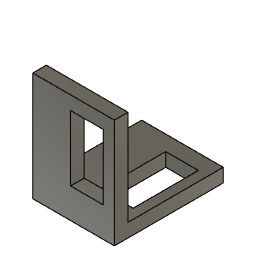
setSquare (Autodesk Fusion 360 design; units mm, degrees)
Autodesk Fusion 360 part; units mm, degrees
sketch "Esquisse1" plane through (0, 0, 0) normal (1, 0, 0) x (0, 1, 0)
  line L0 (0, 0) -> (40, 0)
  line L1 (0, 0) -> (0, 40)
  line L2 (0, 40) -> (5, 40)
  line L3 (5, 40) -> (5, 5)
  line L4 (5, 5) -> (40, 5)
  line L5 (40, 5) -> (40, 0)
  dimension "d2" = 40
  constraint coincident L0.start L1.start
  constraint horizontal L0
  constraint perpendicular L0 L1
  constraint perpendicular L1 L2
  constraint perpendicular L2 L3
  constraint perpendicular L3 L4
  constraint perpendicular L0 L5
  measures "d2" distance of L0.start L0.end
extrude "Extrusion1" add sketch "Esquisse1" along normal blind 30
sketch "Esquisse2" plane through (0, 0, 0) normal (0, 0, 1) x (1, 0, 0)
  line L0 (9.4451, 34.4261) -> (21.4451, 34.4261)
  line L1 (21.4451, 34.4261) -> (21.4451, 10.4261)
  line L2 (21.4451, 10.4261) -> (9.4451, 10.4261)
  line L3 (9.4451, 10.4261) -> (9.4451, 34.4261)
  dimension "d5" = 12
  dimension "d6" = 24
  constraint horizontal L0
  constraint vertical L1
  constraint horizontal L2
  constraint vertical L3
  measures "d5" distance of L0.start L0.end
  measures "d6" distance of L0.end L1.end
extrude "Extrusion2" cut sketch "Esquisse2" along normal blind 6
sketch "Esquisse4" plane through (0, 5, 0) normal (0, 1, 0) x (-1, 0, 0)
  line L0 (0, 5) -> (0, 40)
  line L1 (0, 40) -> (-30, 40)
  line L2 (-30, 40) -> (-30, 5)
  line L3 (-30, 5) -> (0, 5)
  line L4 (-8.8938, 10.999) -> (-20.8938, 10.999)
  line L5 (-20.8938, 10.999) -> (-20.8938, 34.999)
  line L6 (-20.8938, 34.999) -> (-8.8938, 34.999)
  line L7 (-8.8938, 34.999) -> (-8.8938, 10.999)
  dimension "d15" = 12
  dimension "d16" = 24
  constraint horizontal L4
  constraint vertical L5
  constraint horizontal L6
  constraint vertical L7
  measures "d15" distance of L4.start L4.end
  measures "d16" distance of L4.start L6.end
extrude "Extrusion3" cut sketch "Esquisse4" against normal blind 34 contours L4 L5 L6 L7
extrude "Extrusion4" cut 1 faces at (20.8938, 3.3333, 18.999) along direction (1, 0, 0) blind 5
extrude "Extrusion5" add 1 faces at (8.8938, 3.3333, 26.999) along direction (1, 0, 0) blind 5
extrude "Extrusion6" cut 1 faces at (21.4451, 26.4261, 1.6667) along direction (1, 0, 0) blind 5
extrude "Extrusion7" add 1 faces at (9.4451, 18.4261, 1.6667) along direction (1, 0, 0) blind 5
